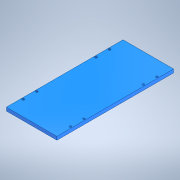
# Autodesk Inventor part: Крышка на отсек с батареей
Saved by Autodesk Inventor 2022 (Build 260153000, 153)
## iProperties
Created: 2021-12-25
Part Number: Крышка на отсек с батареей
Material: Пластик ПЭТ
Document SubType Name: Modeling
Designer: Grigori
Density: 1.541 g/cm^3
Appearance: Поликарбонат — прозрачный
Author: Grigori
Autodesk Inventor part; units mm, degrees
ref_plane "YZ Plane" through (0, 0, 0) normal (1, 0, 0) x (0, 1, 0)
ref_plane "XZ Plane" through (0, 0, 0) normal (0, 1, 0) x (-1, 0, 0)
ref_plane "XY Plane" through (0, 0, 0) normal (0, 0, 1) x (1, 0, 0)
sketch "Эскиз1" plane through (0, 0, 0) normal (0, 1, 0) x (-1, 0, 0)
  line L0 (57.5, 47) -> (132.5, 47)
  line L1 (132.5, 47) -> (132.5, 220)
  line L2 (132.5, 220) -> (57.5, 220)
  line L3 (57.5, 47) -> (57.5, 220)
  circle A0 centre (130, 197.5) radius 1.5
  circle A1 centre (130, 177.5) radius 1.5
  circle A2 centre (130, 69.5) radius 1.5
  circle A3 centre (130, 89.5) radius 1.5
  circle A4 centre (60, 197.5) radius 1.5
  circle A5 centre (60, 177.5) radius 1.5
  circle A6 centre (60, 69.5) radius 1.5
  circle A7 centre (60, 89.5) radius 1.5
  point P0 (0, 0)
  dimension "d10" = 3
  dimension "d11" = 3
  constraints: 8 centre point, 8 end point, 1 horizontal, 1 perpendicular, 1 vertical
  measures "d10" diameter of A0
  measures "d11" diameter of A1
extrude "Выдавливание1" add sketch "Эскиз1" along normal blind 5
